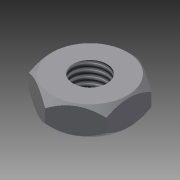
# Autodesk Inventor part: 6-32_Nut
Saved by Autodesk Inventor 2015 (Build 190159000, 159)
## iProperties
Created: 2017-03-10
Part Number: 6-32_Nut
Material: Generic
Document SubType Name: Modeling
Designer: Ernest
Density: 1 g/cm^3
Appearance: Default
Author: Ernest
Autodesk Inventor part; units mm, degrees
ref_plane "YZ Plane" through (0, 0, 0) normal (1, 0, 0) x (0, 1, 0)
ref_plane "XZ Plane" through (0, 0, 0) normal (0, 1, 0) x (-1, 0, 0)
sketch "Sketch1" plane through (0, 0, 0) normal (0, 0, 1) x (1, 0, 0)
  circle A0 centre (0, 0) radius 1.7
  line L0 (0, 4.5207) -> (3.915, 2.2603)
  line L1 (3.915, 2.2603) -> (3.915, -2.2603)
  line L2 (3.915, -2.2603) -> (0, -4.5207)
  line L3 (0, -4.5207) -> (-3.915, -2.2603)
  line L4 (-3.915, -2.2603) -> (-3.915, 2.2603)
  line L5 (-3.915, 2.2603) -> (0, 4.5207)
  dimension "d0" = 3.4
  dimension "d1" = 7.83
  constraints: 12 end point, 2 coincident, 1 centre point, 13 other
  measures "d0" diameter of A0
  measures "d1" distance between parallel lines of L2 L5
extrude "Extrusion1" add sketch "Sketch1" along normal blind 2.83
ref_plane "Work Plane1" through (7.83, 0, 0) normal (0, -1, 0) x (0, 0, -1)
sketch "Sketch2" plane through (7.83, 0, 0) normal (0, -1, 0) x (0, 0, -1)
  line L0 (-4.8262, -6.0526) -> (-1.415, -2.6414)
  line L1 (-1.415, -2.6414) -> (1.5665, -5.6229)
  line L2 (1.5665, -5.6229) -> (3.8499, -3.3395)
  line L3 (3.8499, -3.3395) -> (-1.9469, 2.4574)
  line L4 (-1.9469, 2.4574) -> (-7.6415, -3.2372)
  line L5 (-7.6415, -3.2372) -> (-4.8262, -6.0526)
  line L6 (-2.83, -3.915) -> (-2.83, -7.83) projected
  line L7 (0, -3.915) -> (-2.83, -3.915) projected
  line L8 (0, -7.83) -> (0, -3.915) projected
  line L9 (-2.83, -7.83) -> (0, -7.83)
  line L10 (0, -7.83) -> (-2.83, -7.83) projected
  dimension "d4" = 45
  dimension "d5" = 0.1
  dimension "d6" = 0.1
  constraints: 14 end point, 5 perpendicular, 1 collinear
  measures "d4" angle of L7 L0
  measures "d5" distance from line of L6.start L0
  measures "d6" distance from line of L7.start L1
revolve "Revolution1" cut sketch "Sketch2" angle 360 about axis through (0, 0, 2.83) along (0, 0, -1) contours L5 L4 L3 L2 L1 L8 L7 L0 L6 | L6 L7 L0 | L7 L8 L1
thread "Thread1" size "M3.5x0.6" class "6H" standard "ANSI Metric M Profile" full length
body "Solid1"
